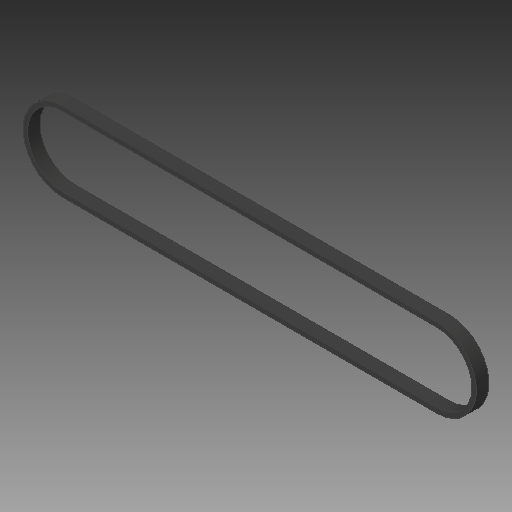
# Autodesk Inventor part: DGB_005_Short Belt_Gates_695-5M-09
Saved by Autodesk Inventor 2018.3 (Build 223284000, 284)
## iProperties
Created: 2020-01-18
Part Number: DGB_005_Short Belt_Gates_695-5M-09
Material: Generic
Document SubType Name: Modeling
Designer: myerpaul
Density: 1 g/cm^3
Appearance: Default
Mass: 20.0624 g
Surface Area: 170.961 cm^2
Volume: 20.0624 cm^3
Author: myerpaul
Autodesk Inventor part; units mm, degrees
ref_plane "YZ Plane" through (0, 0, 0) normal (1, 0, 0) x (0, 1, 0)
ref_plane "XZ Plane" through (0, 0, 0) normal (0, 1, 0) x (-1, 0, 0)
ref_plane "XY Plane" through (0, 0, 0) normal (0, 0, 1) x (1, 0, 0)
sketch "Sketch1" plane through (0, 0, 0) normal (0, 0, 1) x (1, 0, 0)
  circle A0 centre (0, 0) radius 24.892
  circle A1 centre (267.462, 0) radius 24.892
  line L0 (0, 0) -> (267.462, 0) construction
  line L1 (0, -25.019) -> (267.462, -25.019)
  line L2 (267.462, 25.019) -> (0, 25.019)
  arc A2 (0, 25.019) -> (0, -25.019) centre (0, 0) ccw
  arc A3 (267.462, -25.019) -> (267.462, 25.019) centre (267.462, 0) ccw
  line L3 (0, 28.194) -> (267.462, 28.194)
  arc A4 (267.462, -28.194) -> (267.462, 28.194) centre (267.462, 0) ccw
  line L4 (267.462, -28.194) -> (0, -28.194)
  arc A5 (0, 28.194) -> (0, -28.194) centre (0, 0) ccw
  line L5 (7.3323, 0) -> (3.6662, -6.35)
  line L6 (3.6662, -6.35) -> (-3.6662, -6.35)
  line L7 (-3.6662, -6.35) -> (-7.3323, 0)
  line L8 (-7.3323, 0) -> (-3.6662, 6.35)
  line L9 (-3.6662, 6.35) -> (3.6662, 6.35)
  line L10 (3.6662, 6.35) -> (7.3323, 0)
  line L11 (274.7943, 0) -> (271.1282, -6.35)
  line L12 (271.1282, -6.35) -> (263.7958, -6.35)
  line L13 (263.7958, -6.35) -> (260.1297, 0)
  line L14 (260.1297, 0) -> (263.7958, 6.35)
  line L15 (263.7958, 6.35) -> (271.1282, 6.35)
  line L16 (271.1282, 6.35) -> (274.7943, 0)
  point P0 (133.731, 0)
  dimension "d0" = 49.784
  dimension "d1" = 267.462
  dimension "d2" = 3.175
  dimension "d3" = 0.127
  dimension "d8" = 12.7
  constraints: 36 end point, 8 point on circle, 6 centre point, 4 tangent, 3 coincident, 2 parallel, 1 collinear, 1 equal radius, 1 horizontal, 1 horizontal alignment, 1 midpoint, 1 point on line, 29 other
  measures "d0" diameter of A0
  measures "d1" distance of L0.end point (0, 0)
  measures "d2" distance between parallel lines of L3 L2
  measures "d3" radial gap between concentric circles of A3 A1
  measures "d8" distance between parallel lines of L6 L9
extrude "Extrusion2" add sketch "Sketch1" along normal blind 9 contours L3 A4 L4 A5
body "Solid1"
body "Solid2"
